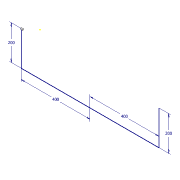
# Autodesk Inventor part: Motor
Saved by Autodesk Inventor 2021 (Build 250183000, 183)
## iProperties
Created: 2021-05-03
Part Number: Motor
Material: Generic
Document SubType Name: Modeling
Designer: Santiago Suárez
Density: 1 g/cm^3
Appearance: Default
Author: Santiago Suárez
Autodesk Inventor part; units mm, degrees
ref_plane "XZ Plane" through (0, 0, 0) normal (0, 1, 0) x (-1, 0, 0)
ref_plane "Work Plane1" through (244.5295, 464.3316, -573.6921) normal (0, 0, 1) x (1, 0, 0)
sketch "Sketch1" plane through (244.5295, 464.3316, -573.6921) normal (0, 0, 1) x (1, 0, 0)
  line L0 (27.0839, -713) -> (65.1217, -713) projected
  line L1 (46.1028, -713) -> (-353.8972, -713)
  line L2 (-353.8972, -713) -> (-353.8972, -513)
  line L3 (46.1028, -713) -> (446.1028, -713)
  line L4 (446.1028, -713) -> (446.1028, -513)
  point P0 (-244.5295, -464.3316)
  dimension "d0" = 400
  dimension "d1" = 200
  dimension "d2" = 400
  dimension "d3" = 200
  constraints: 8 end point, 2 horizontal, 2 perpendicular, 1 midpoint
  measures "d0" distance of L1.start L1.end
  measures "d1" distance of L1.end L2.end
  measures "d2" distance of L1.start L3.end
  measures "d3" distance of L3.end L4.end
ref_plane "Work Plane2" through (-109.5, 0, 0) normal (1, 0, 0) x (0, 1, 0)
sketch "Sketch3" plane through (-109.5, 0, 0) normal (1, 0, 0) x (0, 1, 0)
  line L0 (-48.6684, -573.6921) -> (-48.6684, -548.6921)
  circle A0 centre (-48.6684, -573.6921) radius 5
  point P0 (0, 0)
  dimension "d6" = 25
  dimension "d7" = 10
  constraints: 2 end point, 1 centre point, 1 coincident, 1 vertical
  measures "d6" distance of L0.start L0.end
  measures "d7" diameter of A0
extrude "Extrusion1" add sketch "Sketch3" along normal blind 10
body "Solid1"
